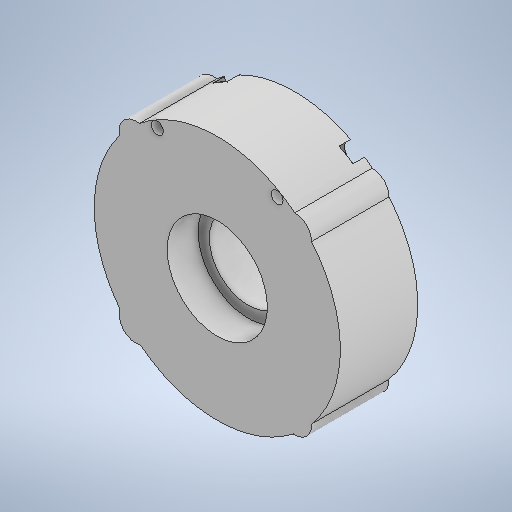
# Autodesk Inventor part: 2024_08_22_LED_blende
Saved by Autodesk Inventor 2025.1 (Build 291241000, 241)
## iProperties
Created: 2023-11-21
Part Number: 2024_08_22_LED_blende
Material: Generisch
Document SubType Name: Modeling
Designer: Daniel
Density: 1 g/cm^3
Appearance: Vorgabe
Author: Daniel
Autodesk Inventor part; units mm, degrees
ref_plane "YZ Plane" through (0, 0, 0) normal (1, 0, 0) x (0, 1, 0)
ref_plane "XZ Plane" through (0, 0, 0) normal (0, 1, 0) x (-1, 0, 0)
ref_plane "XY Plane" through (0, 0, 0) normal (0, 0, 1) x (1, 0, 0)
sketch "Sketch1" plane through (0, 0, 0) normal (0, 0, 1) x (1, 0, 0)
  circle A0 centre (0, 0) radius 11.25
  arc A1 (-32.7929, -17.201) -> (-31.2929, -19.799) centre (0, 0) ccw
  line L0 (-32.7929, -17.201) -> (-31.0547, -16.1974)
  line L1 (-32.7929, -17.201) -> (-31.0547, -16.1974)
  line L2 (-29.5547, -18.7955) -> (-31.2929, -19.799)
  line L3 (-31.2929, -19.799) -> (-29.5547, -18.7955)
  line L4 (-16.1974, -31.0547) -> (-17.201, -32.7929)
  line L5 (-17.201, -32.7929) -> (-16.1974, -31.0547)
  arc A2 (-19.799, -31.2929) -> (-17.201, -32.7929) centre (0, 0) ccw
  line L6 (-19.799, -31.2929) -> (-18.7955, -29.5547)
  line L7 (-19.799, -31.2929) -> (-18.7955, -29.5547)
  arc A3 (17.201, -32.7929) -> (19.799, -31.2929) centre (0, 0) ccw
  line L8 (17.201, -32.7929) -> (16.1974, -31.0547)
  line L9 (17.201, -32.7929) -> (16.1974, -31.0547)
  line L10 (18.7955, -29.5547) -> (19.799, -31.2929)
  line L11 (19.799, -31.2929) -> (18.7955, -29.5547)
  arc A4 (31.2929, -19.799) -> (32.7929, -17.201) centre (0, 0) ccw
  line L12 (31.2929, -19.799) -> (29.5547, -18.7955)
  line L13 (31.0547, -16.1974) -> (32.7929, -17.201)
  line L14 (32.7929, -17.201) -> (31.0547, -16.1974)
  line L15 (32.7929, 17.201) -> (31.0547, 16.1974)
  line L16 (32.7929, 17.201) -> (31.0547, 16.1974)
  arc A5 (32.7929, 17.201) -> (31.2929, 19.799) centre (0, 0) ccw
  line L17 (29.5547, 18.7955) -> (31.2929, 19.799)
  line L18 (31.2929, 19.799) -> (29.5547, 18.7955)
  line L19 (16.1974, 31.0547) -> (17.201, 32.7929)
  line L20 (17.201, 32.7929) -> (16.1974, 31.0547)
  line L21 (19.799, 31.2929) -> (18.7955, 29.5547)
  line L22 (19.799, 31.2929) -> (18.7955, 29.5547)
  line L23 (-17.201, 32.7929) -> (-16.1974, 31.0547)
  line L24 (-17.201, 32.7929) -> (-16.1974, 31.0547)
  line L25 (-18.7955, 29.5547) -> (-19.799, 31.2929)
  line L26 (-19.799, 31.2929) -> (-18.7955, 29.5547)
  arc A6 (-31.2615, 19.7809) -> (-32.7929, 17.201) centre (-0.5443, -0.1969) ccw
  line L27 (-31.2615, 19.7809) -> (-29.5547, 18.7955)
  line L28 (-31.2615, 19.7809) -> (-29.5547, 18.7955)
  line L29 (-31.0547, 16.1974) -> (-32.7929, 17.201)
  line L30 (-32.7929, 17.201) -> (-31.0547, 16.1974)
  arc A7 (-27.9532, 21.6091) -> (-22.3503, 27.212) centre (-22.995, 22.2538) ccw
  circle A8 centre (-22.995, 22.2538) radius 5
  circle A9 centre (21.9063, 22.2538) radius 5
  circle A10 centre (21.9063, 22.2538) radius 5
  circle A11 centre (-22.995, 22.2538) radius 4.75
  circle A12 centre (-22.995, -22.6475) radius 4.75
  circle A13 centre (21.9063, -22.6475) radius 4.75
  circle A14 centre (21.9063, 22.2538) radius 4.75
  circle A15 centre (0, 0) radius 34.775
  circle A16 centre (0, 0) radius 36.75
  point P0 (0, 0)
  point P1 (0, 49.75)
  point P2 (26.6556, 22.3333)
  point P3 (21.9111, 27.0038)
  point P4 (-22.0321, 26.9051)
  point P5 (-27.6123, 21.1391)
  point P6 (-27.5325, -21.2429)
  point P7 (-21.6596, -27.2059)
  point P8 (21.4454, -27.3751)
  point P9 (26.6466, -22.3441)
  dimension "d6" = 70.05
  dimension "d8" = 74.0608
  dimension "d0" = 10
  dimension "d1" = 0.25
  dimension "d4" = 360
  dimension "d7" = 0.25
  dimension "d9" = 73.5
  constraints: 62 end point, 17 centre point, 15 collinear, 14 point on circle, 8 coincident, 8 other
  measures "d0" diameter of A8
  measures "d1" radial gap between concentric circles of A8 A11
  measures "d9" diameter of A16
extrude "Extrusion1" add sketch "Sketch1" along normal blind 21.9 contours A0 | A16 A12 | A12 A15 A16 | A15 A7 A9 A13 A12 | A12 A15 | A15 A11 A7 | A11 A15 | A15 A11 | A15 A13 | A13 A15 | A15 A14 A9 | A15 A14 | A14 A15 picked at (20.2713, 26.7736)
sketch "Skizze4" plane through (0, 0, 21.9) normal (0, 0, 1) x (1, 0, 0)
  circle A0 centre (0, 0) radius 11
  dimension "d24" = 22
  constraints: 1 centre point, 1 coincident
  measures "d24" diameter of A0
extrude "Extrusion4" cut sketch "Skizze4" against normal up to surface (21.9 mm away) from surface at 0
sketch "Skizze5" plane through (0, 0, 21.9) normal (0, 0, 1) x (1, 0, 0)
  circle A0 centre (0, 0) radius 11 projected
  circle A1 centre (0, 0) radius 14.17
  dimension "d27" = 28.34
  constraints: 1 centre point, 1 coincident
  measures "d27" diameter of A1
extrude "Extrusion5" cut sketch "Skizze5" against normal blind 8.76 contours A0 | A1
sketch "Skizze6" plane through (0, 0, 0) normal (0, 0, -1) x (-1, 0, 0)
  line L0 (0, 0) -> (-16.92, 0)
  line L1 (-16.92, 0) -> (-16.92, 28.34)
  line L2 (-16.92, 28.34) -> (0, 28.34)
  line L3 (0, 28.34) -> (0, 0)
  circle A0 centre (-16.92, 28.34) radius 1.7
  circle A1 centre (16.92, 28.34) radius 1.7
  dimension "d30" = 16.92
  dimension "d31" = 28.34
  dimension "d32" = 3.4
  constraints: 8 end point, 2 centre point, 2 coincident, 2 parallel, 2 symmetric about line, 1 horizontal, 1 perpendicular, 1 other
  measures "d30" distance from line of L3 L1.end
  measures "d31" distance between parallel lines of L0 L2
  measures "d32" diameter of A0
extrude "Extrusion6" cut sketch "Skizze6" against normal through all contours A0 L2 L1 | L1 L2 A0 | A1
sketch "Skizze8" plane through (0, 0, 0) normal (0, 0, -1) x (-1, 0, 0)
  circle A0 centre (-16.92, 28.34) radius 1.7 projected
  circle A1 centre (-16.92, 28.34) radius 2.855
  circle A2 centre (16.92, 28.34) radius 1.7 projected
  circle A3 centre (16.92, 28.34) radius 2.855
  point P0 (0, 0)
  dimension "d39" = 5.71
  dimension "d40" = 5.71
  constraints: 4 coincident, 2 centre point
  measures "d39" diameter of A1
  measures "d40" diameter of A3
extrude "Extrusion8" cut sketch "Skizze8" against normal blind 3.29 contours A1 | A2 | A3
body "Solid1"
